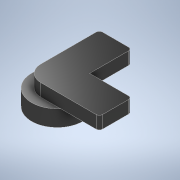
# Autodesk Inventor part: Door Lock
Saved by Autodesk Inventor 2021 (Build 250183000, 183)
## iProperties
Created: 2020-08-11
Part Number: Door Lock
Material: Generic
Document SubType Name: Modeling
Designer: jgray
Density: 1 g/cm^3
Appearance: Glossy - Black
Author: jgray
Autodesk Inventor part; units mm, degrees
ref_plane "YZ Plane" through (0, 0, 0) normal (1, 0, 0) x (0, 1, 0)
ref_plane "XZ Plane" through (0, 0, 0) normal (0, 1, 0) x (-1, 0, 0)
ref_plane "XY Plane" through (0, 0, 0) normal (0, 0, 1) x (1, 0, 0)
sketch "Sketch1" plane through (0, 0, 0) normal (0, 1, 0) x (-1, 0, 0)
  circle A0 centre (0, 0) radius 15.75
  dimension "d0" = 31.5
  constraints: 1 centre point, 1 coincident
  measures "d0" diameter of A0
extrude "Extrusion1" add sketch "Sketch1" along normal blind 10
sketch "Sketch2" plane through (0, 10, 0) normal (0, 1, 0) x (1, 0, 0)
  circle A0 centre (0, 0) radius 10
  line L0 (0, -10) -> (34, -10)
  line L1 (-10, 0) -> (-10, 34)
  line L2 (0, 10) -> (34, 10)
  line L3 (10, 0) -> (10, 34)
  line L4 (-8, 36) -> (8, 36)
  line L5 (36, -8) -> (36, 8)
  arc A1 (34, -10) -> (36, -8) centre (34, -8) ccw
  arc A2 (36, 8) -> (34, 10) centre (34, 8) ccw
  arc A3 (10, 34) -> (8, 36) centre (8, 34) ccw
  arc A4 (-8, 36) -> (-10, 34) centre (-8, 34) ccw
  point P0 (36, -10)
  point P1 (-10, 36)
  point P2 (10, 10)
  dimension "d3" = 20
  dimension "d4" = 36
  dimension "d5" = 36
  dimension "d6" = 2
  dimension "d7" = 20
  dimension "d8" = 20
  constraints: 12 end point, 12 point on circle, 9 tangent, 5 centre point, 4 point on line, 3 equal radius, 2 horizontal, 2 perpendicular, 2 vertical, 1 coincident
  measures "d3" diameter of A0
  measures "d4" horizontal distance of point (36, -10) point (0, 0)
  measures "d5" vertical distance of point (-10, 36) point (0, 0)
  measures "d6" radius of A1
  measures "d7" distance between parallel lines of L0 L2
  measures "d8" distance between parallel lines of L1 L3
extrude "Extrusion2" add sketch "Sketch2" along normal blind 7.8
body "Solid1"
